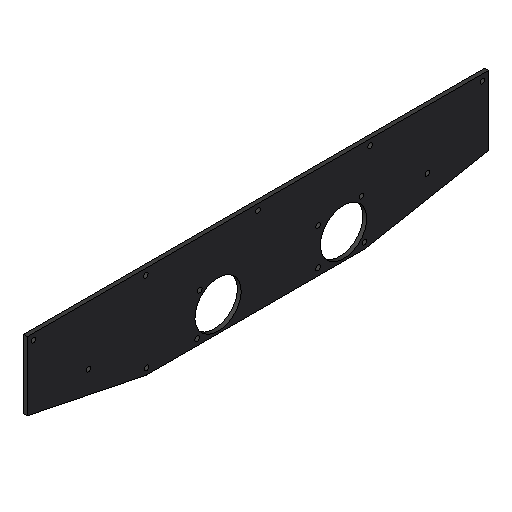
# Autodesk Inventor part: ChassiInsidePlate3.3
Saved by Autodesk Inventor 2023 (Build 270158000, 158)
## iProperties
Created: 2022-11-07
Part Number: ChassiInsidePlate3.3
Material: Generic
Document SubType Name: Modeling
Designer: deli
Density: 1 g/cm^3
Appearance: Default
Author: deli
Autodesk Inventor part; units mm, degrees
ref_plane "YZ Plane" through (0, 0, 0) normal (1, 0, 0) x (0, 1, 0)
ref_plane "XZ Plane" through (0, 0, 0) normal (0, 1, 0) x (-1, 0, 0)
ref_plane "XY Plane" through (0, 0, 0) normal (0, 0, 1) x (1, 0, 0)
sketch "Sketch1" plane through (0, 0, 0) normal (1, 0, 0) x (0, 1, 0)
  arc A0 (526.028, -141.2971) -> (524.9794, -138.6702) centre (524.1903, -140.5079) ccw projected
  arc A1 (218.0959, -5.5727) -> (219.3067, -7.4104) centre (220.0959, -5.5727) ccw projected
  line L0 (218.0959, -5.5727) -> (218.0959, 225.8641) projected
  line L1 (218.0959, 225.8641) -> (133.9428, 225.8641) projected
  line L2 (133.9428, 225.8641) -> (114.1971, 129.252) projected
  arc A2 (114.1971, 129.252) -> (114.0959, 128.2508) centre (119.0959, 128.2508) ccw projected
  arc A3 (114.0959, -50.2813) -> (114.1833, -51.2122) centre (119.0959, -50.2813) ccw projected
  line L3 (114.1833, -51.2122) -> (133.2497, -151.8359) projected
  line L4 (133.2497, -151.8359) -> (217.4027, -151.8359) projected
  circle A4 centre (185.0959, -146.8359) radius 2 projected
  circle A5 centre (185.0959, 128.9391) radius 2 projected
  circle A6 centre (152.5266, 84.772) radius 2 projected
  circle A7 centre (153.0149, -47.6855) radius 2 projected
  circle A8 centre (142.0959, 175.8641) radius 2 projected
  circle A9 centre (142.0959, -101.8359) radius 2 projected
  circle A10 centre (134.8459, 69.6739) radius 7 projected
  circle A11 centre (134.8459, -33.1787) radius 7 projected
  circle A12 centre (149.8506, -12.2522) radius 2 projected
  circle A13 centre (119.8411, -12.2522) radius 2 projected
  circle A14 centre (119.0959, 86.7765) radius 2 projected
  circle A15 centre (185.0959, 220.8641) radius 2 projected
  circle A16 centre (185.0959, -54.9109) radius 2 projected
  circle A17 centre (185.0959, 37.0141) radius 2 projected
  circle A18 centre (119.0959, 128.2508) radius 2 projected
  circle A19 centre (119.0959, -50.2813) radius 2 projected
  line L5 (190.0959, 225.8641) -> (190.0959, -151.8359)
  circle A20 centre (134.8459, 69.6739) radius 19
  circle A21 centre (134.8459, -33.1787) radius 19
  line L6 (524.9794, -138.6702) -> (506.3839, -130.685) projected
  line L7 (114.0959, 128.2508) -> (114.0959, -50.2813) projected
  line L8 (217.4027, -151.8359) -> (524.0551, -145.8914) projected
  line L9 (524.0551, -145.8914) -> (526.028, -141.2971) projected
  circle A22 centre (256.6682, -27.263) radius 1 projected
  circle A23 centre (339.366, -62.7745) radius 1 projected
  circle A24 centre (435.8468, -104.2046) radius 1 projected
  circle A25 centre (518.5446, -139.7161) radius 1 projected
  arc A26 (503.8869, -124.4298) -> (506.3839, -130.685) centre (508.263, -126.3089) ccw projected
  line L10 (503.8869, -124.4298) -> (507.7005, -115.5488) projected
  arc A27 (507.7005, -115.5488) -> (502.1873, -113.1814) centre (504.9439, -114.3651) ccw projected
  line L11 (502.1873, -113.1814) -> (498.3737, -122.0623) projected
  arc A28 (492.1185, -124.5593) -> (498.3737, -122.0623) centre (493.9977, -120.1832) ccw projected
  line L12 (492.1185, -124.5593) -> (219.3067, -7.4104) projected
  circle A29 centre (504.9439, -114.3651) radius 1.5 projected
  circle A30 centre (200.5959, 173.6641) radius 1.6 projected
  circle A31 centre (215.5959, 163.6641) radius 1.6 projected
  circle A32 centre (215.5959, 192.5641) radius 1.6 projected
  circle A33 centre (200.5959, 202.5641) radius 1.6 projected
  circle A34 centre (215.5959, 202.5641) radius 1.6 projected
  circle A35 centre (200.5959, 192.5641) radius 1.6 projected
  circle A36 centre (215.5959, 173.6641) radius 1.6 projected
  circle A37 centre (200.5959, 163.6641) radius 1.6 projected
  point P0 (0, 0)
  point P1 (114.0959, 111.4062)
  dimension "d0" = 5
  dimension "d1" = 38
  dimension "d2" = 38
  constraints: 2 centre point, 2 coincident, 2 end point, 2 point on line, 1 vertical
  measures "d0" distance from line of L5 A5.centre
  measures "d1" diameter of A20
  measures "d2" diameter of A21
extrude "Extrusion1" add sketch "Sketch1" along normal blind 3.175 contours L4 L3 A3 L7 A2 L2 L1 L5
body "Solid1"
